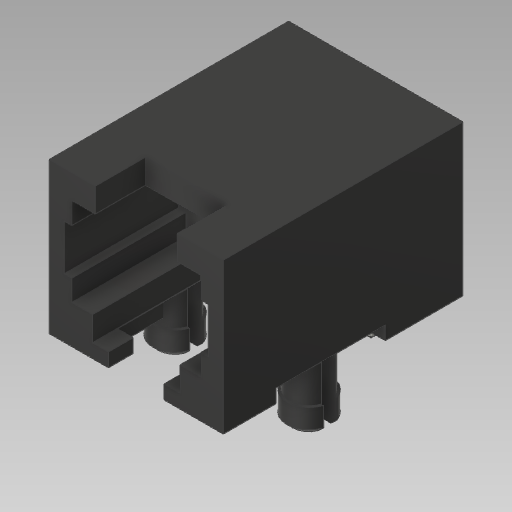
# Autodesk Inventor part: RJ12 - 90deg
Saved by Autodesk Inventor 2020 (Build 240168000, 168)
## iProperties
Created: 2017-10-30
Part Number: RJ12 - 90deg
Material: Thermoplastic Resin
Document SubType Name: Modeling
Designer: Alex
Mass: 2.45784 g
Surface Area: 14.2326 cm^2
Volume: 1.92018 cm^3
Density: 1.28 g/cm^3
Appearance: Smooth - Black
Author: Alex
Autodesk Inventor part; units mm, degrees
ref_plane "XZ Plane" through (0, 0, 0) normal (0, 1, 0) x (-1, 0, 0)
sketch "Sketch1" plane through (0, 0, 0) normal (0, 0, 1) x (1, 0, 0)
  line L0 (6.604, -5.715) -> (-6.604, -5.715)
  line L1 (-6.604, -5.715) -> (-6.604, 5.715)
  line L2 (-6.604, 5.715) -> (6.604, 5.715)
  line L3 (6.604, 5.715) -> (6.604, -5.715)
  line L4 (6.604, -5.715) -> (-6.604, 5.715) construction
  line L5 (-6.604, -5.715) -> (6.604, 5.715) construction
  point P0 (0, 0)
  dimension "d0" = 13.208
  dimension "d1" = 11.43
  constraints: 12 end point, 2 midpoint, 2 parallel, 1 horizontal, 1 perpendicular
  measures "d0" distance of L1.end L2.end
  measures "d1" distance of L0.end L1.end
extrude "Extrusion1" add sketch "Sketch1" along normal mid plane 18.161
sketch "Sketch2" plane through (0, 0, 9.0805) normal (0, 0, 1) x (1, 0, 0)
  line L0 (0, -4.6736) -> (-3.3147, -4.6736)
  line L1 (-3.3147, -4.6736) -> (-3.3147, -2.8194)
  line L2 (-3.3147, -2.8194) -> (-4.8895, -2.8194)
  line L3 (-4.8895, -2.8194) -> (-4.8895, -1.2192)
  line L4 (-4.8895, -1.2192) -> (-5.461, -1.2192)
  line L5 (-5.461, -1.2192) -> (-5.461, 2.2352)
  line L6 (-5.461, 2.2352) -> (-4.8895, 2.2352)
  line L7 (-4.8895, 2.2352) -> (-4.8895, 3.8735)
  line L8 (-4.8895, 3.8735) -> (0, 3.8735)
  line L9 (0, 3.8735) -> (0, -4.6736) construction
  line L10 (6.604, 5.715) -> (-6.604, 5.715) construction
  line L11 (-6.604, -5.715) -> (6.604, -5.715) construction
  line L12 (0, -4.6736) -> (3.3147, -4.6736)
  line L13 (3.3147, -4.6736) -> (3.3147, -2.8194)
  line L14 (3.3147, -2.8194) -> (4.8895, -2.8194)
  line L15 (4.8895, -2.8194) -> (4.8895, -1.2192)
  line L16 (4.8895, -1.2192) -> (5.461, -1.2192)
  line L17 (5.461, -1.2192) -> (5.461, 2.2352)
  line L18 (5.461, 2.2352) -> (4.8895, 2.2352)
  line L19 (4.8895, 2.2352) -> (4.8895, 3.8735)
  line L20 (4.8895, 3.8735) -> (0, 3.8735)
  point P0 (0, 0)
  dimension "d17" = 1.8415
  dimension "d18" = 4.8895
  dimension "d19" = 5.461
  dimension "d20" = 1.0414
  dimension "d21" = 1.8542
  dimension "d22" = 4.4958
  dimension "d23" = 3.4798
  dimension "d24" = 3.3147
  constraints: 38 end point, 8 symmetric about line, 7 perpendicular, 5 point on line, 1 horizontal, 1 vertical, 1 other
  measures "d17" distance between parallel lines of L10 L8
  measures "d18" distance between parallel lines of L9 L7
  measures "d19" distance between parallel lines of L9 L5
  measures "d20" distance between parallel lines of L11 L0
  measures "d21" distance of L0.end L1.end
  measures "d22" distance between parallel lines of L11 L4
  measures "d23" distance between parallel lines of L10 L6
  measures "d24" distance between parallel lines of L9 L1
extrude "Extrusion2" cut sketch "Sketch2" against normal blind 8.6614
sketch "Sketch3" plane through (-6.604, 5.715, 9.0805) normal (0, 1, 0) x (1, 0, 0)
  line L0 (3.4925, 0) -> (9.7155, 0)
  line L1 (9.7155, 0) -> (9.7155, 3.81)
  line L2 (9.7155, 3.81) -> (3.4925, 3.81)
  line L3 (3.4925, 3.81) -> (3.4925, 0)
  line L4 (13.208, 0) -> (0, 0) projected
  point P0 (6.604, 9.0805)
  point P1 (6.604, 3.81)
  dimension "d27" = 6.223
  dimension "d28" = 3.81
  constraints: 8 end point, 2 parallel, 1 horizontal, 1 midpoint, 1 perpendicular, 1 point on line, 1 vertical alignment
  measures "d27" distance of L1.end L2.end
  measures "d28" distance of L0.end L1.end
extrude "Extrusion3" cut sketch "Sketch3" against normal up to surface (1.8415 mm away)
sketch "Sketch4" plane through (-6.604, -5.715, 9.0805) normal (0, -1, 0) x (1, 0, 0)
  line L0 (9.9187, 0) -> (3.2893, 0) projected
  line L1 (4.4958, 0) -> (4.4958, -1.8669)
  line L2 (4.4958, -1.8669) -> (3.3147, -1.8669)
  line L3 (3.3147, -1.8669) -> (3.3147, -10.9347)
  line L4 (3.3147, -10.9347) -> (9.8933, -10.9347)
  line L5 (9.8933, -10.9347) -> (9.8933, -1.8669)
  line L6 (9.8933, -1.8669) -> (8.7122, -1.8669)
  line L7 (8.7122, -1.8669) -> (8.7122, 0)
  line L8 (8.7122, 0) -> (4.4958, 0)
  point P0 (6.604, -9.0805)
  point P1 (6.604, 0)
  point P2 (6.604, -10.9347)
  dimension "d31" = 1.8669
  dimension "d32" = 4.2164
  dimension "d33" = 9.0678
  dimension "d34" = 6.5786
  constraints: 16 end point, 4 perpendicular, 3 point on line, 3 vertical alignment, 2 midpoint, 1 parallel, 1 vertical
  measures "d31" distance of L1.start L1.end
  measures "d32" distance between parallel lines of L7 L1
  measures "d33" distance of L4.end L5.end
  measures "d34" distance between parallel lines of L3 L5
extrude "Extrusion4" cut sketch "Sketch4" against normal up to surface (1.0414 mm away)
sketch "Sketch5" plane through (-6.604, -5.715, -9.0805) normal (0, -1, 0) x (1, 0, 0)
  line L0 (0, 18.161) -> (0, 0) projected
  line L1 (0, 14.1605) -> (1.1176, 14.1605)
  line L2 (1.1176, 14.1605) -> (1.1176, 12.8143)
  line L3 (1.1176, 12.8143) -> (3.3147, 12.8143)
  line L4 (3.3147, 12.8143) -> (3.3147, 7.2263)
  line L5 (3.3147, 7.2263) -> (1.1176, 7.2263)
  line L6 (1.1176, 7.2263) -> (1.1176, 5.8801)
  line L7 (1.1176, 5.8801) -> (0, 5.8801)
  line L8 (0, 5.8801) -> (0, 14.1605)
  line L9 (3.3147, 7.2263) -> (3.3147, 16.2941) construction
  line L10 (6.604, 9.0805) -> (6.604, 17.5857) construction
  line L11 (1.3335, 1.3716) -> (1.3335, 5.8674)
  line L12 (1.3335, 5.8674) -> (11.8745, 5.8674)
  line L13 (11.8745, 5.8674) -> (11.8745, 1.3716)
  line L14 (11.8745, 1.3716) -> (10.7315, 1.3716)
  line L15 (10.7315, 1.3716) -> (10.7315, 4.7244)
  line L16 (10.7315, 4.7244) -> (2.4765, 4.7244)
  line L17 (2.4765, 4.7244) -> (2.4765, 1.3716)
  line L18 (2.4765, 1.3716) -> (1.3335, 1.3716)
  line L19 (13.208, 0) -> (0, 0) projected
  line L20 (13.208, 14.1605) -> (12.0904, 14.1605)
  line L21 (12.0904, 14.1605) -> (12.0904, 12.8143)
  line L22 (12.0904, 12.8143) -> (9.8933, 12.8143)
  line L23 (9.8933, 12.8143) -> (9.8933, 7.2263)
  line L24 (9.8933, 7.2263) -> (12.0904, 7.2263)
  line L25 (12.0904, 7.2263) -> (12.0904, 5.8801)
  line L26 (12.0904, 5.8801) -> (13.208, 5.8801)
  line L27 (13.208, 5.8801) -> (13.208, 14.1605)
  point P0 (6.604, 5.8674)
  dimension "d38" = 5.588
  dimension "d39" = 1.1176
  dimension "d41" = 8.2804
  dimension "d42" = 1.143
  dimension "d43" = 4.4958
  dimension "d44" = 1.143
  dimension "d45" = 1.3716
  dimension "d46" = 10.541
  constraints: 50 end point, 11 perpendicular, 8 symmetric about line, 7 point on line, 2 collinear, 2 vertical, 1 horizontal, 1 midpoint, 1 vertical alignment
  measures "d38" distance between parallel lines of L5 L3
  measures "d39" distance of L1.start L1.end
  measures "d41" distance between parallel lines of L7 L1
  measures "d42" distance between parallel lines of L16 L12
  measures "d43" distance between parallel lines of L12 L14
  measures "d44" distance between parallel lines of L13 L15
  measures "d45" distance between parallel lines of L19 L14
  measures "d46" distance between parallel lines of L13 L11
extrude "Extrusion5" cut sketch "Sketch5" against normal blind 1.016
ref_plane "Work Plane1" through (5.08, 0, 0) normal (1, 0, 0) x (0, 1, 0)
ref_plane "Work Plane2" through (-5.08, 0, 0) normal (1, 0, 0) x (0, 1, 0)
sketch "Sketch6" plane through (5.08, 0, 0) normal (1, 0, 0) x (0, 1, 0)
  line L0 (-4.6736, 2.5781) -> (-7.5565, 2.5781)
  line L1 (-7.5565, 2.5781) -> (-7.5565, 2.7305)
  line L2 (-7.5565, 2.7305) -> (-9.0297, 2.7305)
  line L3 (-9.0297, 2.7305) -> (-9.4361, 2.3241)
  line L4 (-9.4361, 2.3241) -> (-9.4361, 1.0541)
  line L5 (-9.4361, 1.0541) -> (-4.6736, 1.0541)
  line L6 (-4.6736, 2.5781) -> (-4.6736, 1.0541)
  line L7 (-4.6736, 9.0805) -> (-4.6736, 0.4191) construction
  line L8 (-4.6736, 9.0805) -> (-5.715, 9.0805) construction
  point P0 (0, 0)
  point P1 (0, 0)
  dimension "d51" = 1.524
  dimension "d53" = 1.6764
  dimension "d54" = 45
  dimension "d55" = 1.27
  dimension "d58" = 4.7625
  dimension "d59" = 1.4732
  dimension "d60" = 6.5024
  constraints: 15 end point, 3 perpendicular, 1 parallel, 1 point on line
  measures "d51" distance between parallel lines of L5 L0
  measures "d53" distance between parallel lines of L5 L2
  measures "d54" angle of L2 L3
  measures "d55" distance from line of L5 L3.end
  measures "d58" distance between parallel lines of L4 L6
  measures "d59" distance of L1.end L2.end
  measures "d60" distance between parallel lines of L8 L0
revolve "Revolution1" add sketch "Sketch6" angle 360 about axis through (5.08, -9.4361, 1.0541) along (0, 1, 0)
sketch "Sketch7" plane through (-5.08, 0, 0) normal (1, 0, 0) x (0, 1, 0)
  line L0 (-4.6736, 2.5781) -> (-7.5565, 2.5781)
  line L1 (-7.5565, 2.5781) -> (-7.5565, 2.7305)
  line L2 (-7.5565, 2.7305) -> (-9.0297, 2.7305)
  line L3 (-9.0297, 2.7305) -> (-9.4361, 2.3241)
  line L4 (-9.4361, 2.3241) -> (-9.4361, 1.0541)
  line L5 (-9.4361, 1.0541) -> (-4.6736, 1.0541)
  line L6 (-4.6736, 2.5781) -> (-4.6736, 1.0541)
  line L7 (-4.6736, 9.0805) -> (-4.6736, 0.4191) construction
  line L8 (-4.6736, 9.0805) -> (-5.715, 9.0805) construction
  point P0 (0, 0)
  point P1 (0, 0)
  point P2 (0, 0)
  dimension "d62" = 1.524
  dimension "d63" = 1.6764
  dimension "d64" = 45
  dimension "d65" = 1.27
  dimension "d66" = 4.7625
  dimension "d67" = 1.4732
  dimension "d68" = 6.5024
  constraints: 19 end point, 3 perpendicular, 1 parallel, 1 point on line
  measures "d62" distance between parallel lines of L5 L0
  measures "d63" distance between parallel lines of L5 L2
  measures "d64" angle of L2 L3
  measures "d65" distance from line of L5 L3.end
  measures "d66" distance between parallel lines of L4 L6
  measures "d67" distance of L1.end L2.end
  measures "d68" distance between parallel lines of L8 L0
revolve "Revolution2" add sketch "Sketch7" angle 360 about axis through (-5.08, -9.4361, 1.0541) along (0, 1, 0)
sketch "Sketch8" plane through (-5.08, -9.4361, 1.0541) normal (0, -1, 0) x (1, 0, 0)
  line L0 (-1.6764, 0.4953) -> (11.8364, 0.4953)
  line L1 (11.8364, 0.4953) -> (11.8364, -0.4953)
  line L2 (11.8364, -0.4953) -> (-1.6764, -0.4953)
  line L3 (-1.6764, -0.4953) -> (-1.6764, 0.4953)
  circle A0 centre (0, 0) radius 1.6764 construction
  circle A1 centre (10.16, 0) radius 1.6764 construction
  point P0 (5.08, -1.0541)
  point P1 (-1.6764, 0)
  point P2 (11.8364, 0)
  dimension "d70" = 0.9906
  constraints: 8 end point, 3 horizontal alignment, 2 midpoint, 2 parallel, 1 horizontal, 1 perpendicular, 2 other
  measures "d70" distance between parallel lines of L2 L0
extrude "Extrusion6" cut sketch "Sketch8" against normal up to surface (4.7371 mm away)
sketch "Sketch9" plane through (-6.604, -5.715, -9.0805) normal (0, -1, 0) x (1, 0, 0)
  line L0 (9.7155, 14.351) -> (3.4925, 14.351)
  line L1 (9.7155, 18.161) -> (9.7155, 14.351)
  line L2 (3.4925, 14.351) -> (3.4925, 18.161)
  circle A0 centre (9.906, 3.6576) radius 0.3175
  circle A1 centre (8.636, 1.1176) radius 0.3175
  line L3 (9.7155, 14.351) -> (3.4925, 14.351) projected
  line L4 (13.208, 0) -> (13.208, 5.8801) projected
  line L5 (13.208, 0) -> (0, 0) projected
  circle A2 centre (7.366, 3.6576) radius 0.3175
  circle A3 centre (6.096, 1.1176) radius 0.3175
  circle A4 centre (4.826, 3.6576) radius 0.3175
  circle A5 centre (3.556, 1.1176) radius 0.3175
  point P0 (6.604, 9.0805)
  dimension "d73" = 3.302
  dimension "d74" = 2.54
  dimension "d75" = 1.27
  dimension "d76" = 3.6576
  dimension "d77" = 0.635
  dimension "d80" = 2.54
  constraints: 6 centre point, 6 end point, 1 equal radius, 1 horizontal, 8 other
  measures "d73" distance from line of L4 A0.centre
  measures "d74" vertical distance of A1.centre A0.centre
  measures "d75" horizontal distance of A1.centre A0.centre
  measures "d76" distance from line of L5 A0.centre
  measures "d77" diameter of A0
  measures "d80" distance of A0.centre A2.centre
extrude "Extrusion7" add sketch "Sketch9" along normal blind 2.54 and the other way blind 1.27
chamfer "Chamfer1" distance 0.254 angle 45 6 edges at (1.7145, -8.255, -7.9629) (2.9845, -8.255, -5.4229) (0.4445, -8.255, -5.4229) (-0.8255, -8.255, -7.9629) (-2.0955, -8.255, -5.4229) (-3.3655, -8.255, -7.9629)
equation "\"d44\" = d42"
equation "\"d50\" = -d49"
equation "\"d49\" = 5.08"
body "Solid1"
